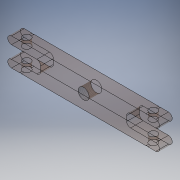
# Autodesk Inventor part: ハンド_ピストン先
Saved by Autodesk Inventor 2019.4 (Build 234330000, 330)
## iProperties
Created: 2021-12-05
Part Number: ハンド_ピストン先
Material: ポリカーボネート、スモーク
Document SubType Name: Modeling
Designer: 堀川皓史
Density: 1.2 g/cm^3
Appearance: ポリカーボネート - スモーク
Mass: 29.1068 g
Surface Area: 56.736 cm^2
Volume: 10.7803 cm^3
Author: 堀川皓史
Autodesk Inventor part; units mm, degrees
ref_plane "YZ Plane" through (0, 0, 0) normal (1, 0, 0) x (0, 1, 0)
ref_plane "XZ Plane" through (0, 0, 0) normal (0, 1, 0) x (-1, 0, 0)
ref_plane "XY Plane" through (0, 0, 0) normal (0, 0, 1) x (1, 0, 0)
sketch "スケッチ1" plane through (0, 0, 0) normal (0, 0, 1) x (1, 0, 0)
  circle A0 centre (0, 0) radius 5 construction
  line L0 (-60, 11) -> (-50.7483, 11)
  line L1 (60, 11) -> (60, 5)
  line L2 (60, 5) -> (34, 5)
  line L3 (34, 5) -> (34, -5)
  line L4 (34, -5) -> (60, -5)
  line L5 (60, -5) -> (60, -11)
  line L6 (60, -11) -> (50.7483, -11)
  line L7 (-60, -11) -> (-60, -5)
  line L8 (-60, -5) -> (-34, -5)
  line L9 (-34, -5) -> (-34, 5)
  line L10 (-34, 5) -> (-60, 5)
  line L11 (-60, 5) -> (-60, 11)
  arc A1 (-49.2517, 11) -> (-50.7483, 11) centre (-50, 12.3) ccw construction
  arc A2 (50.7483, 11) -> (49.2517, 11) centre (50, 12.3) ccw construction
  arc A3 (-50.7483, -11) -> (-49.2517, -11) centre (-50, -12.3) ccw construction
  arc A4 (49.2517, -11) -> (50.7483, -11) centre (50, -12.3) ccw construction
  arc A5 (-50.7483, 11) -> (-49.2517, 11) centre (-50, 12.3) ccw
  line L12 (-49.2517, 11) -> (49.2517, 11)
  line L13 (-50.7483, 11) -> (-49.2517, 11) construction
  line L14 (-49.2517, -11) -> (-50.7483, -11) construction
  line L15 (-50.7483, -11) -> (-60, -11)
  arc A6 (-49.2517, -11) -> (-50.7483, -11) centre (-50, -12.3) ccw
  arc A7 (49.2517, 11) -> (50.7483, 11) centre (50, 12.3) ccw
  line L16 (50.7483, 11) -> (60, 11)
  line L17 (49.2517, 11) -> (50.7483, 11) construction
  arc A8 (50.7483, -11) -> (49.2517, -11) centre (50, -12.3) ccw
  line L18 (50.7483, -11) -> (49.2517, -11) construction
  line L19 (49.2517, -11) -> (-49.2517, -11)
  dimension "d0" = 10
  dimension "d1" = 10
  dimension "d2" = 10
  dimension "d3" = 5
  dimension "d4" = 5
  dimension "d5" = 6
  dimension "d6" = 6
  dimension "d7" = 3
  dimension "d8" = 3
  dimension "d9" = 3
  dimension "d10" = 3
  dimension "d11" = 1.3
  dimension "d12" = 1.3
  dimension "d13" = 1.3
  dimension "d14" = 1.3
  dimension "d15" = 100
  dimension "d17" = 50
  dimension "d19" = 16
  dimension "d20" = 10
  dimension "d21" = 10
  dimension "d22" = 16
  constraints: 40 end point, 22 perpendicular, 16 point on circle, 9 centre point, 5 horizontal, 5 parallel, 4 vertical alignment, 1 coincident, 1 point on line
  measures "d0" diameter of A0
  measures "d1" distance between parallel lines of L4 L2
  measures "d2" distance between parallel lines of L8 L10
  measures "d3" distance from line of point (0, 0) L10
  measures "d4" distance from line of point (0, 0) L2
  measures "d5" distance between parallel lines of L10 L0
  measures "d6" distance between parallel lines of L6 L8
  measures "d7" diameter of A1
  measures "d8" diameter of A2
  measures "d9" diameter of A3
  measures "d10" diameter of A4
  measures "d11" distance from line of L0 A1.centre
  measures "d12" distance from line of L0 A2.centre
  measures "d13" distance from line of A3.centre L6
  measures "d14" distance from line of A4.centre L6
  measures "d15" distance of A2.centre A1.centre
  measures "d17" horizontal distance of point (0, 0) A1.centre
  measures "d19" distance from line of L3 A2.centre
  measures "d20" distance from line of A1.centre L11
  measures "d21" distance from line of A2.centre L1
  measures "d22" distance from line of L9 A1.centre
extrude "押し出し1" add sketch "スケッチ1" along normal blind 10
sketch "スケッチ2" plane through (-49.2517, 11, 0) normal (0, 1, 0) x (1, 0, 0)
  circle A0 centre (-0.7483, -5) radius 3.05
  circle A1 centre (99.2517, -5) radius 3.05
  line L0 (-10.7483, 0) -> (-10.7483, -10) projected
  point P0 (49.2517, 0)
  point P1 (-10.7483, -5)
  dimension "d26" = 6.1
  dimension "d27" = 6.1
  dimension "d28" = 50
  dimension "d29" = 50
  constraints: 2 centre point, 2 horizontal alignment, 1 midpoint
  measures "d26" diameter of A0
  measures "d27" diameter of A1
  measures "d28" horizontal distance of point (49.252, 0) A0.centre
  measures "d29" horizontal distance of point (49.252, 0) A1.centre
extrude "押し出し2" cut sketch "スケッチ2" against normal through all
fillet "フィレット1" radius 3 12 edges at (-34, 5, 5) (-34, -5, 5) (34, 5, 5) (34, -5, 5) (-60, 11, 5) (-60, 5, 5) (-60, -5, 5) (-60, -11, 5) (60, 11, 5) (60, 5, 5) (60, -5, 5) (60, -11, 5)
sketch "スケッチ4" plane through (0, 0, 10) normal (0, 0, 1) x (1, 0, 0)
  point P0 (0, 0)
hole "穴1" at (0, 0, 10) direction (0, 0, -1) diameter 8.647 end through all thread size "M10x1.25" class "6H" standard "ANSI Metric M Profile"
equation "\"d17\" = 0.5 * d15"
